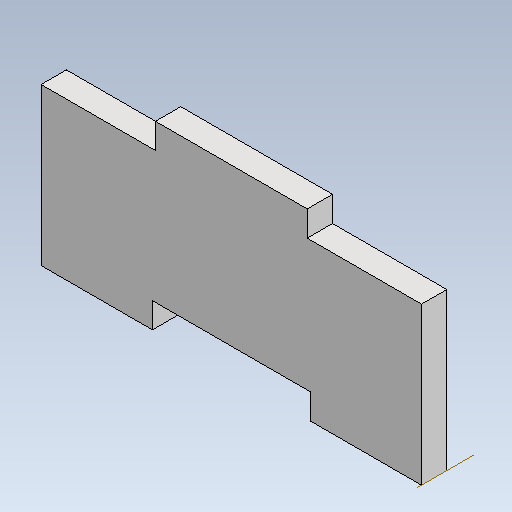
# Autodesk Inventor part: lower-back-plate-support
Saved by Autodesk Inventor 2025 (Build 290162000, 162)
## iProperties
Created: 2025-08-21
Part Number: lower-back-plate-support
Material: Generic
Document SubType Name: Modeling
Designer: HP
Density: 1 g/cm^3
Appearance: Default
Author: HP
Autodesk Inventor part; units mm, degrees
ref_plane "YZ Plane" through (0, 0, 0) normal (1, 0, 0) x (0, 1, 0)
ref_plane "XZ Plane" through (0, 0, 0) normal (0, 1, 0) x (-1, 0, 0)
ref_plane "XY Plane" through (0, 0, 0) normal (0, 0, 1) x (1, 0, 0)
sketch "Sketch1" plane through (0, 0, 0) normal (0, 0, 1) x (1, 0, 0)
  line L0 (-37.6, -18) -> (37.6, -18)
  line L1 (37.6, -18) -> (37.6, 18)
  line L2 (37.6, 18) -> (-37.6, 18)
  line L3 (-37.6, 18) -> (-37.6, -18)
  line L4 (-37.6, -18) -> (37.6, 18) construction
  line L5 (37.6, -18) -> (-37.6, 18) construction
  line L6 (-15.1, 18) -> (5.2739, 18)
  line L7 (-14.8, -18) -> (-37.6, -18)
  line L8 (-37.6, -18) -> (-37.6, -13)
  line L9 (0, 0) -> (0, -18) construction
  line L10 (14.8, -18) -> (37.6, -18)
  line L11 (37.6, -18) -> (37.6, -13)
  line L12 (-15.1, 18) -> (-37.6, 18)
  line L13 (-37.6, 18) -> (-37.6, 13)
  line L14 (15.1, 18) -> (37.6, 18)
  line L15 (37.6, 18) -> (37.6, 13)
  line L16 (-15, -13) -> (15, -13) construction
  line L17 (15, -13) -> (15, -18)
  line L18 (15, -18) -> (-15, -18)
  line L19 (-15, -18) -> (-15, -13)
  line L20 (-15, -13) -> (15, -18) construction
  line L21 (15, -13) -> (-15, -18) construction
  line L22 (-15, -13) -> (-37.6, -13)
  line L23 (15, -13) -> (37.6, -13)
  line L24 (-37.6, 13) -> (-15.6, 13) construction
  line L25 (-15.6, 13) -> (-15.6, 18)
  line L26 (-15.6, 18) -> (-37.6, 18)
  line L27 (-37.6, 18) -> (-37.6, 13)
  line L28 (-37.6, 13) -> (-15.6, 18) construction
  line L29 (-15.6, 13) -> (-37.6, 18) construction
  line L30 (15.6, 13) -> (37.6, 13) construction
  line L31 (37.6, 13) -> (37.6, 18)
  line L32 (37.6, 18) -> (15.6, 18)
  line L33 (15.6, 18) -> (15.6, 13)
  line L34 (15.6, 13) -> (37.6, 18) construction
  line L35 (37.6, 13) -> (15.6, 18) construction
  line L36 (-15.6, 13) -> (15.6, 13)
  point P0 (0, -15.5)
  point P1 (-37.6, -13)
  point P2 (-15, -18)
  point P3 (-26.6, 15.5)
  point P4 (26.6, 15.5)
  point P5 (15.6, 18)
  dimension "d1" = 36
  dimension "d27" = 5
  dimension "d28" = 30
  dimension "d30" = 5
  dimension "d31" = 5
  dimension "d32" = 22
  dimension "d33" = 22
  dimension "d34" = 53.2
  constraints: 74 end point, 10 collinear, 9 equal length, 9 midpoint, 7 horizontal, 7 perpendicular, 1 vertical alignment
  measures "d1" distance between parallel lines of L0 L2
  measures "d27" distance between parallel lines of L16 L18
  measures "d28" distance between parallel lines of L17 L19
  measures "d30" distance between parallel lines of L26 L24
  measures "d31" distance between parallel lines of L32 L30
  measures "d32" distance between parallel lines of L25 L27
  measures "d33" distance between parallel lines of L31 L33
  measures "d34" distance of point (26.6, 15.5) point (-26.6, 15.5)
extrude "Extrusion1" add sketch "Sketch1" along normal blind 5 contours L19 L22 L3 L2 L25 L36 L33 L1 L23 L17 L0
equation "\"d31\" = d30"
equation "\"d33\" = d32"
body "Solid1"
